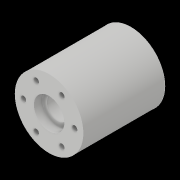
# Autodesk Inventor part: S3_ph
Saved by Autodesk Inventor 2018 (Build 220112000, 112)
## iProperties
Created: 2022-03-24
Part Number: S3_ph
Material: Generic
Document SubType Name: Modeling
Designer: kumpu
Density: 1 g/cm^3
Appearance: Default
Author: kumpu
Autodesk Inventor part; units mm, degrees
ref_plane "YZ Plane" through (0, 0, 0) normal (1, 0, 0) x (0, 1, 0)
ref_plane "XZ Plane" through (0, 0, 0) normal (0, 1, 0) x (-1, 0, 0)
ref_plane "XY Plane" through (0, 0, 0) normal (0, 0, 1) x (1, 0, 0)
sketch "Sketch1" plane through (0, 0, 0) normal (1, 0, 0) x (0, 1, 0)
  line L0 (31.75, 0) -> (14.2875, 0)
  line L1 (14.2875, 0) -> (14.2875, -8.001)
  line L2 (14.2875, -8.001) -> (10.16, -8.001)
  line L3 (10.16, -8.001) -> (10.16, -76.2)
  line L4 (10.16, -76.2) -> (31.75, -76.2)
  line L5 (31.75, -76.2) -> (31.75, 0)
  line L6 (0, 0) -> (0, -76.2)
  dimension "d0" = 63.5
  dimension "d1" = 76.2
  dimension "d2" = 28.575
  dimension "d3" = 8.001
  dimension "d4" = 20.32
  constraints: 14 end point, 5 perpendicular, 2 point on line, 1 coincident, 1 horizontal, 1 vertical
  measures "d0" diameter of L5 L6
  measures "d1" distance of L4.end L0.start
  measures "d2" diameter of L1 L6
  measures "d3" distance of L0.end L1.end
  measures "d4" diameter of L3 L6
revolve "Revolution1" add sketch "Sketch1" angle 360 about axis through (0, 0, 0) along (0, 0, -1)
sketch "Sketch2" plane through (0, 0, 0) normal (0, 0, 1) x (1, 0, 0)
  line L0 (0, 0) -> (-23.8252, 0) construction
  point P0 (-11.9126, -20.6332)
  point P1 (-11.9126, -20.6332)
  point P2 (11.9126, -20.6332)
  point P3 (11.9126, -20.6332)
  point P4 (23.8252, 0)
  point P5 (23.8252, 0)
  point P6 (11.9126, 20.6332)
  point P7 (11.9126, 20.6332)
  point P8 (-11.9126, 20.6332)
  point P9 (-11.9126, 20.6332)
  dimension "d6" = 23.8252
  dimension "d9" = 360
  constraints: 6 coincident, 2 end point, 1 horizontal, 13 other
  measures "d6" distance of L0.start L0.end
hole "Hole1" at (-23.8252, 0, 0) at (-11.9126, -20.6332, 0) at (11.9126, -20.6332, 0) at (23.8252, 0, 0) at (11.9126, 20.6332, 0) at (-11.9126, 20.6332, 0) direction (0, 0, -1) diameter 5 end through all
body "Solid1"
